Autodesk Fusion 360 part; units mm, degrees
(part 4 of 5)
  spline S564 degree 3 poles (63.6009, -62.117) (63.5452, -62.1873) (63.4918, -62.2601) (63.4399, -62.3343) (63.4147, -62.3703) (63.3907, -62.4074) (63.3664, -62.4443) (63.3253, -62.5068) (63.2844, -62.5696) (63.2459, -62.6346) (63.2219, -62.6752) (63.1997, -62.7175) (63.1767, -62.7591) (63.1472, -62.8123) (63.1177, -62.8655) (63.0898, -62.9203) (63.0665, -62.9662) (63.0447, -63.0135) (63.0226, -63.0606) (62.9975, -63.1139) (62.9727, -63.1675) (62.9491, -63.2223) (62.928, -63.2715) (62.9077, -63.3215) (62.8877, -63.3719) (62.8656, -63.4276) (62.8443, -63.4839) (62.8237, -63.541) (62.8052, -63.5925) (62.787, -63.6442) (62.7696, -63.6968) (62.75, -63.7563) (62.7315, -63.8169) (62.7134, -63.8779) (62.6978, -63.9304) (62.6821, -63.9828) (62.6676, -64.0364) (62.6498, -64.1023) (62.6337, -64.1699) (62.6177, -64.2374) (62.6055, -64.2884) (62.5926, -64.3387) (62.5815, -64.3906) (62.5635, -64.4745) (62.5478, -64.5606) (62.5323, -64.6468) knots 516 516 516 516 517 517 517 518 518 518 519 519 519 520 520 520 521 521 521 522 522 522 523 523 523 524 524 524 525 525 525 526 526 526 527 527 527 528 528 528 529 529 529 530 530 530 531 531 531 531
  spline S565 degree 3 poles (62.5323, -64.6468) (62.5253, -64.6848) (62.5171, -64.7216) (62.5105, -64.76) (62.4896, -64.8838) (62.4713, -65.0101) (62.4555, -65.1388) knots 531 531 531 531 532 532 532 533 533 533 533
  spline S566 degree 3 poles (62.4555, -65.1388) (62.4498, -65.1844) (62.4459, -65.2317) (62.4409, -65.2779) (62.4315, -65.3648) (62.4223, -65.4519) (62.4152, -65.541) (62.4107, -65.5971) (62.4076, -65.6547) (62.404, -65.7118) (62.4004, -65.769) (62.3956, -65.8251) (62.3929, -65.8832) knots 533 533 533 533 534 534 534 535 535 535 536 536 536 537 537 537 537
  spline S567 degree 3 poles (62.3929, -65.8832) (60.929, -65.0924) (59.2396, -64.7303) (57.6027, -64.3796) (57.0063, -64.2518) (56.4429, -64.1311) (55.8865, -63.9902) (53.8629, -63.4779) (52.3936, -62.8929) (51.1226, -62.0932) (50.698, -61.826) (50.2974, -61.5052) (49.8733, -61.1654) (49.4956, -60.8629) (49.1052, -60.5501) (48.6984, -60.2812) knots 537 537 537 537 538 538 538 539 539 539 540 540 540 541 541 541 542 542 542 542
  spline S568 degree 3 poles (48.6984, -60.2812) (48.112, -59.6879) (47.5333, -59.0646) (46.9735, -58.4616) (46.4472, -57.8948) (45.9032, -57.3085) (45.3521, -56.7472) (45.2642, -56.6576) (45.1756, -56.5693) (45.0868, -56.4809) knots 542 542 542 542 543 543 543 544 544 544 545 545 545 545
  line L80 (45.0868, -56.4809) -> (45.0182, -56.4139)
  spline S569 degree 3 poles (45.0182, -56.4139) (44.6949, -56.0962) (44.3697, -55.7813) (44.0447, -55.4664) (43.215, -54.6625) (42.357, -53.8314) (41.5512, -52.9714) knots 546 546 546 546 547 547 547 548 548 548 548
  line L81 (41.5512, -52.9714) -> (41.5003, -52.9185)
  spline S570 degree 3 poles (41.5003, -52.9185) (41.4832, -52.9013) (41.4663, -52.884) (41.4498, -52.8662) knots 549 549 549 549 550 550 550 550
  spline S571 degree 3 poles (41.4498, -52.8662) (40.8528, -52.2243) (40.2539, -51.5635) (39.6747, -50.9244) knots 550 550 550 550 551 551 551 551
  line L82 (39.6747, -50.9244) -> (39.2528, -50.4591)
  spline S572 degree 3 poles (39.2528, -50.4591) (39.2451, -50.451) (38.4952, -49.6609) (37.6236, -48.7686) knots 552 552 552 552 553 553 553 553
  line L83 (37.6236, -48.7686) -> (37.6335, -48.7479)
  spline S573 degree 3 poles (37.6335, -48.7479) (37.6362, -48.7422) (37.6387, -48.7366) (37.6415, -48.7309) knots 554 554 554 554 555 555 555 555
  line L84 (37.6415, -48.7309) -> (37.6464, -48.7205)
  spline S574 degree 3 poles (37.6464, -48.7205) (37.7592, -48.4837) (37.8712, -48.2488) (37.9778, -48.0153) knots 556 556 556 556 557 557 557 557
  spline S575 degree 3 poles (37.9778, -48.0153) (38.4446, -46.9908) (38.9842, -45.9631) (39.6279, -44.8736) (39.7256, -44.7081) (39.8268, -44.5413) (39.9304, -44.3732) (39.9626, -44.3209) (39.9966, -44.2678) (40.0294, -44.2152) (40.1022, -44.0987) (40.1756, -43.9818) (40.2514, -43.8637) (40.2926, -43.7995) (40.3355, -43.7343) (40.3776, -43.6696) (40.4483, -43.5611) (40.5196, -43.4521) (40.593, -43.342) (40.6394, -43.2723) (40.687, -43.2017) (40.7346, -43.1313) (40.8076, -43.0232) (40.8818, -42.9144) (40.9576, -42.8046) (41.0074, -42.7324) (41.0578, -42.6597) (41.1088, -42.5866) (41.1873, -42.4743) (41.2677, -42.3606) (41.3491, -42.2463) (41.4006, -42.1739) (41.452, -42.1016) (41.5048, -42.0282) (41.5924, -41.9065) (41.6829, -41.7827) (41.7741, -41.6583) (41.824, -41.5902) (41.8729, -41.5229) (41.9239, -41.4539) (42.0361, -41.3024) (42.152, -41.1479) (42.2696, -40.992) (42.3028, -40.9481) (42.3343, -40.9055) (42.3678, -40.8612) (42.3733, -40.854) (42.3793, -40.8464) (42.3847, -40.8392) knots 557 557 557 557 558 558 558 559 559 559 560 560 560 561 561 561 562 562 562 563 563 563 564 564 564 565 565 565 566 566 566 567 567 567 568 568 568 569 569 569 570 570 570 571 571 571 572 572 572 573 573 573 573
  spline S576 degree 3 poles (42.3847, -40.8392) (42.3816, -40.8575) (42.3797, -40.876) (42.3766, -40.8943) (42.3477, -41.0657) (42.3222, -41.2377) (42.301, -41.4103) knots 573 573 573 573 574 574 574 575 575 575 575
  spline S577 degree 3 poles (42.301, -41.4103) (42.2993, -41.4247) (42.297, -41.439) (42.2953, -41.4534) knots 575 575 575 575 576 576 576 576
  spline S578 degree 3 poles (42.2953, -41.4534) (42.2741, -41.632) (42.2583, -41.8113) (42.2454, -41.991) (42.243, -42.025) (42.2403, -42.059) (42.2381, -42.0931) (42.2272, -42.2674) (42.2204, -42.4419) (42.2172, -42.6167) (42.2166, -42.6524) (42.2164, -42.6881) (42.2161, -42.7238) knots 576 576 576 576 577 577 577 578 578 578 579 579 579 580 580 580 580
  spline S579 degree 3 poles (42.2161, -42.7238) (42.2146, -42.9023) (42.2161, -43.0809) (42.2227, -43.2596) (42.2235, -43.2795) (42.2249, -43.2994) (42.2257, -43.3194) knots 580 580 580 580 581 581 581 582 582 582 582
  spline S580 degree 3 poles (42.2257, -43.3194) (42.233, -43.491) (42.2442, -43.6625) (42.2589, -43.8339) (42.2612, -43.8603) (42.2629, -43.8868) (42.2654, -43.9132) (42.2817, -44.0896) (42.3029, -44.2657) (42.3272, -44.4415) (42.3323, -44.4781) (42.3374, -44.5148) (42.3428, -44.5514) (42.3687, -44.726) (42.3981, -44.9001) (42.4318, -45.0736) (42.4377, -45.1045) (42.4444, -45.1352) (42.4506, -45.166) knots 582 582 582 582 583 583 583 584 584 584 585 585 585 586 586 586 587 587 587 588 588 588 588
  spline S581 degree 3 poles (42.4506, -45.166) (42.4876, -45.3485) (42.5276, -45.5306) (42.5733, -45.7116) knots 588 588 588 588 589 589 589 589
  ellipse E72 centre (56.6932, -41.7046) end of major axis (43.7029, -48.5965) minor radius 14.1081 (42.5733, -45.7116) -> (43.5329, -48.2653) ccw
  line L85 (43.5329, -48.2653) -> (43.592, -48.3797)
  ellipse E73 centre (53.8644, -44.6888) end of major axis (43.8869, -37.796) minor radius 10.4203 (43.592, -48.3797) -> (45.426, -51.0359) ccw
  spline S582 degree 3 poles (45.426, -51.0359) (49.4743, -55.6013) (55.686, -55.4114) (59.19, -54.8409) knots 592 592 592 592 593 593 593 593
  ellipse E74 centre (57.3687, -53.9917) end of major axis (58.3854, -55.9418) minor radius 1.7755 (58.8424, -55.5685) -> (59.19, -54.8409) ccw
  spline S583 degree 3 poles (58.8424, -55.5685) (58.7415, -55.6913) (58.4247, -56.1135) (58.5847, -56.3946) knots 594 594 594 594 595 595 595 595
  spline S584 degree 3 poles (58.5847, -56.3946) (58.6701, -56.545) (58.8483, -56.6007) (59.1137, -56.5599) (59.6558, -56.4764) (60.4864, -55.9417) (60.6187, -55.8147) knots 595 595 595 595 596 596 596 597 597 597 597
  spline S585 degree 3 poles (60.6187, -55.8147) (60.6941, -55.7415) (60.7615, -55.6603) (60.8219, -55.569) knots 597 597 597 597 598 598 598 598
  spline S586 degree 3 poles (60.8219, -55.569) (61.9106, -56.1881) (63.4433, -56.428) (64.404, -55.5311) knots 598 598 598 598 599 599 599 599
  spline S587 degree 3 poles (64.404, -55.5311) (64.5308, -55.413) (64.5814, -55.2388) (64.5394, -55.065) (64.4963, -54.8868) (64.3637, -54.7461) (64.1931, -54.6977) knots 599 599 599 599 600 600 600 601 601 601 601
  line L86 (64.1931, -54.6977) -> (64.1043, -54.6725)
  spline S588 degree 3 poles (64.1043, -54.6725) (63.4425, -54.485) (62.8117, -54.3065) (62.2722, -53.9865) knots 602 602 602 602 603 603 603 603
  spline S589 degree 3 poles (62.2722, -53.9865) (65.482, -52.7483) (70.6811, -49.8991) (71.9549, -44.1657) knots 603 603 603 603 604 604 604 604
  ellipse E75 centre (60.8257, -42.7322) end of major axis (67.3496, -31.9795) minor radius 11.0029 (71.9549, -44.1657) -> (72.2688, -40.9515) ccw
  line L87 (72.2688, -40.9515) -> (72.2641, -40.8116)
  ellipse E76 centre (64.0549, -39.8245) end of major axis (61.025, -29.7414) minor radius 7.9821 (72.2641, -40.8116) -> (71.864, -38.1233) ccw
  spline S590 degree 3 poles (71.864, -38.1233) (71.3093, -36.0365) (70.2055, -34.159) (68.6718, -32.6934) (66.8596, -30.9618) (64.5325, -29.8716) (61.9419, -29.5414) (61.4484, -29.4785) (60.9282, -29.4355) (60.3894, -29.4131) knots 607 607 607 607 608 608 608 609 609 609 610 610 610 610
  spline S591 degree 3 poles (60.3894, -29.4131) (62.1442, -28.8512) (63.6979, -28.4325) (65.1254, -28.1369) (66.5537, -27.841) (67.8818, -27.634) (69.1854, -27.505) (69.4822, -27.4757) (69.783, -27.4409) (70.086, -27.4058) (70.2077, -27.3917) (70.33, -27.3777) (70.4526, -27.3638) (70.5356, -27.3544) (70.6189, -27.3455) (70.7022, -27.3365) (70.7407, -27.3324) (70.779, -27.328) (70.8175, -27.3239) (71.0588, -27.2986) (71.3009, -27.2759) (71.5425, -27.2581) knots 610 610 610 610 611 611 611 612 612 612 613 613 613 614 614 614 615 615 615 616 616 616 617 617 617 617
  spline S592 degree 3 poles (71.5425, -27.2581) (71.546, -27.2578) (71.5495, -27.2575) (71.5529, -27.2572) knots 617 617 617 617 618 618 618 618
  spline S593 degree 3 poles (71.5529, -27.2572) (71.6573, -27.2496) (71.7614, -27.2435) (71.8655, -27.238) (71.8846, -27.237) (71.9037, -27.2355) (71.9227, -27.2346) (72.011, -27.2303) (72.0988, -27.2279) (72.1867, -27.2255) (72.222, -27.2245) (72.2575, -27.2227) (72.2928, -27.2221) (72.3654, -27.2208) (72.4375, -27.2216) (72.5098, -27.2218) (72.5604, -27.2219) (72.6112, -27.2211) (72.6617, -27.222) (72.7198, -27.2231) (72.7774, -27.2263) (72.8352, -27.2286) (72.8911, -27.2307) (72.9472, -27.2324) (73.0028, -27.2357) knots 618 618 618 618 619 619 619 620 620 620 621 621 621 622 622 622 623 623 623 624 624 624 625 625 625 626 626 626 626
  spline S594 degree 3 poles (73.0028, -27.2357) (73.1238, -27.2975) (73.2558, -27.3369) (73.3903, -27.3647) knots 626 626 626 626 627 627 627 627
  spline S595 degree 3 poles (73.3903, -27.3647) (73.3976, -27.3661) (73.4048, -27.3679) (73.412, -27.3693) knots 627 627 627 627 628 628 628 628
  spline S596 degree 3 poles (73.412, -27.3693) (73.4649, -27.3796) (73.5178, -27.3883) (73.5709, -27.3953) (73.5825, -27.3968) (73.594, -27.3989) (73.6056, -27.4003) (73.6624, -27.4071) (73.719, -27.4127) (73.7748, -27.417) (74.7297, -27.4916) (75.7369, -27.313) (76.5412, -26.9278) (77.045, -26.6866) (77.529, -26.3489) (77.9038, -25.9766) (78.1899, -25.6923) (78.1926, -25.1937) (77.9094, -24.8875) knots 628 628 628 628 629 629 629 630 630 630 631 631 631 632 632 632 633 633 633 634 634 634 634
  spline S597 degree 3 poles (77.9094, -24.8875) (77.5689, -24.5207) (77.0072, -24.5165) (76.597, -24.5137) (76.5457, -24.5133) (76.4961, -24.513) (76.4487, -24.5119) knots 634 634 634 634 635 635 635 636 636 636 636
  spline S598 degree 3 poles (76.4487, -24.5119) (76.366, -24.5102) (76.283, -24.5097) (76.1996, -24.509) knots 636 636 636 636 637 637 637 637
  spline S599 degree 3 poles (76.1996, -24.509) (75.7309, -24.5056) (75.2883, -24.5023) (74.8824, -24.3113) (74.8326, -24.2878) (74.8004, -24.2682) (74.7801, -24.2534) knots 637 637 637 637 638 638 638 639 639 639 639
  spline S600 degree 3 poles (74.7801, -24.2534) (74.8118, -24.232) (74.8678, -24.2024) (74.9585, -24.171) (75.4633, -23.9965) (75.9971, -24.0882) (76.4053, -24.1876) (76.515, -24.2143) (76.6253, -24.2575) (76.7421, -24.3032) (76.9584, -24.3877) (77.1762, -24.4768) (77.4332, -24.4704) knots 639 639 639 639 640 640 640 641 641 641 642 642 642 643 643 643 643
  spline S601 degree 3 poles (77.4332, -24.4704) (77.6931, -24.4651) (77.9655, -24.3065) (78.0953, -24.0844) (78.2126, -23.8837) (78.2118, -23.6512) (78.0931, -23.4295) (77.584, -22.4789) (76.7066, -22.0668) (75.9993, -21.8141) (75.9082, -21.7815) (75.8143, -21.7464) (75.718, -21.7106) (75.6611, -21.6894) (75.6027, -21.6677) (75.5439, -21.646) knots 643 643 643 643 644 644 644 645 645 645 646 646 646 647 647 647 648 648 648 648
  spline S602 degree 3 poles (75.5439, -21.646) (75.5305, -21.6411) (75.5172, -21.6363) (75.5037, -21.6314) (75.4494, -21.6115) (75.3942, -21.5917) (75.3384, -21.5721) (75.3288, -21.5687) (75.3194, -21.5654) (75.3098, -21.562) knots 648 648 648 648 649 649 649 650 650 650 651 651 651 651
  spline S603 degree 3 poles (75.3098, -21.562) (75.2458, -21.5398) (75.181, -21.5181) (75.1155, -21.4971) (75.1056, -21.4939) (75.0956, -21.491) (75.0856, -21.4878) (75.0302, -21.4704) (74.9744, -21.4537) (74.9181, -21.4377) (74.9031, -21.4335) (74.8881, -21.4292) (74.873, -21.4251) (74.7411, -21.3889) (74.6074, -21.3581) (74.473, -21.3352) (74.4574, -21.3326) (74.4419, -21.3303) (74.4264, -21.3279) (74.3698, -21.3191) (74.3132, -21.3119) (74.2567, -21.3064) (74.2447, -21.3052) (74.2327, -21.3036) (74.2207, -21.3026) (74.1534, -21.2969) (74.0861, -21.2937) (74.019, -21.2935) (74.0157, -21.2935) (74.0124, -21.293) (74.0091, -21.293) (73.9985, -21.293) (73.9881, -21.2942) (73.9775, -21.2944) (73.9331, -21.295) (73.8887, -21.2967) (73.8445, -21.3001) (73.8254, -21.3015) (73.8063, -21.3036) (73.7872, -21.3056) (73.7475, -21.3098) (73.708, -21.3152) (73.6687, -21.3218) (73.6485, -21.3252) (73.6284, -21.3286) (73.6083, -21.3327) (73.5685, -21.3408) (73.5288, -21.3508) (73.4893, -21.3617) (73.4713, -21.3667) (73.4531, -21.3709) (73.4351, -21.3765) (73.3817, -21.3932) (73.3287, -21.4123) (73.2763, -21.4347) (73.2732, -21.436) (73.2701, -21.4367) (73.267, -21.4381) knots 651 651 651 651 652 652 652 653 653 653 654 654 654 655 655 655 656 656 656 657 657 657 658 658 658 659 659 659 660 660 660 661 661 661 662 662 662 663 663 663 664 664 664 665 665 665 666 666 666 667 667 667 668 668 668 669 669 669 670 670 670 670
  spline S604 degree 3 poles (73.267, -21.4381) (73.2211, -21.4583) (73.1773, -21.4804) (73.1351, -21.5046) knots 670 670 670 670 671 671 671 671
  spline S605 degree 3 poles (73.1351, -21.5046) (73.0842, -21.4915) (73.0305, -21.4797) (72.9785, -21.4671) (72.9191, -21.4527) (72.8604, -21.438) (72.7996, -21.4243) (72.734, -21.4096) (72.6664, -21.396) (72.5992, -21.3821) (72.5352, -21.3688) (72.4719, -21.3552) (72.4066, -21.3428) (72.3399, -21.33) (72.2713, -21.3184) (72.2032, -21.3064) (72.1348, -21.2944) (72.0669, -21.282) (71.9971, -21.2708) (71.9297, -21.2599) (71.8604, -21.2501) (71.7917, -21.2399) (71.7184, -21.2291) (71.6457, -21.2179) (71.571, -21.2079) (71.5034, -21.1988) (71.4341, -21.1908) (71.3654, -21.1823) (71.2874, -21.1727) (71.2098, -21.1629) (71.1304, -21.1541) (71.0627, -21.1466) (70.9934, -21.1401) (70.9247, -21.1333) (70.8419, -21.125) (70.7595, -21.1164) (70.6753, -21.109) (70.6076, -21.103) (70.5382, -21.0979) (70.4696, -21.0925) (70.3826, -21.0855) (70.296, -21.0784) (70.2078, -21.0723) (70.1399, -21.0677) (70.0707, -21.0639) (70.0021, -21.0598) (69.9107, -21.0543) (69.8196, -21.0485) (69.7269, -21.0438) (69.6603, -21.0405) (69.5923, -21.038) (69.525, -21.0351) (69.4287, -21.0309) (69.3327, -21.0265) (69.2351, -21.0233) (69.1686, -21.021) (69.101, -21.0196) (69.0339, -21.0178) (68.934, -21.0151) (68.8344, -21.0122) (68.7333, -21.0104) (68.6667, -21.0092) (68.5991, -21.0088) (68.532, -21.008) (68.4289, -21.0067) (68.326, -21.0053) (68.2218, -21.0049) (68.1555, -21.0046) (68.0882, -21.0052) (68.0215, -21.0053) (67.915, -21.0055) (67.8086, -21.0055) (67.7011, -21.0066) (67.6353, -21.0072) (67.5687, -21.0086) (67.5026, -21.0096) (67.3931, -21.0112) (67.2838, -21.0126) (67.1733, -21.0151) (67.1074, -21.0166) (67.0408, -21.0188) (66.9746, -21.0206) (66.8626, -21.0236) (66.7507, -21.0264) (66.6379, -21.0303) (66.5728, -21.0325) (66.5071, -21.0354) (66.4418, -21.0379) (66.3271, -21.0423) (66.2126, -21.0466) (66.0972, -21.0518) (66.0317, -21.0548) (65.9656, -21.0584) (65.8998, -21.0616) (65.7836, -21.0673) (65.6675, -21.0729) (65.5507, -21.0794) (65.4858, -21.0831) (65.4205, -21.0873) (65.3554, -21.0912) (65.2373, -21.0982) (65.1192, -21.1051) (65.0005, -21.1129) (64.9342, -21.1173) (64.8675, -21.1223) (64.801, -21.1269) (64.6832, -21.1351) (64.5654, -21.1431) (64.4472, -21.152) (64.3812, -21.1569) (64.315, -21.1625) (64.2489, -21.1677) (64.1292, -21.1771) (64.0096, -21.1864) (63.8897, -21.1965) (63.8234, -21.2021) (63.7569, -21.2083) (63.6905, -21.2141) (63.5718, -21.2245) (63.4531, -21.2347) (63.3343, -21.2458) (63.2606, -21.2527) (63.1868, -21.2601) (63.1131, -21.2673) (63.0004, -21.2781) (62.8878, -21.2888) (62.7751, -21.3002) (62.7033, -21.3075) (62.6315, -21.3154) (62.5597, -21.3229) (62.4451, -21.3349) (62.3305, -21.3467) (62.216, -21.3592) (62.1434, -21.3672) (62.071, -21.3757) (61.9984, -21.3838) (61.8854, -21.3966) (61.7724, -21.4091) (61.6596, -21.4224) (61.5783, -21.4319) (61.4974, -21.442) (61.4162, -21.4518) (61.3125, -21.4643) (61.2087, -21.4766) (61.1052, -21.4895) (61.0166, -21.5006) (60.9284, -21.5123) (60.8401, -21.5236) (60.7441, -21.536) (60.648, -21.548) (60.5523, -21.5607) (60.4622, -21.5727) (60.3727, -21.5851) (60.2829, -21.5973) (60.1895, -21.61) (60.0958, -21.6225) (60.0028, -21.6355) (59.9108, -21.6484) (59.8195, -21.6617) (59.7279, -21.6749) (59.6379, -21.6878) (59.5475, -21.7004) (59.4579, -21.7136) (59.3548, -21.7288) (59.2526, -21.7444) (59.1501, -21.7599) (59.0734, -21.7715) (58.9962, -21.7828) (58.9199, -21.7945) (58.8058, -21.8121) (58.6929, -21.8302) (58.5798, -21.8481) (58.5154, -21.8583) (58.4503, -21.8683) (58.3862, -21.8786) (58.2765, -21.8963) (58.1682, -21.9144) (58.0595, -21.9324) (57.9929, -21.9434) (57.9256, -21.9542) (57.8593, -21.9653) (57.7345, -21.9863) (57.6112, -22.0077) (57.4879, -22.0291) (57.4394, -22.0375) (57.3901, -22.0457) (57.3419, -22.0541) (57.1705, -22.0842) (57.0007, -22.1145) (56.8325, -22.1452) knots 671 671 671 671 672 672 672 673 673 673 674 674 674 675 675 675 676 676 676 677 677 677 678 678 678 679 679 679 680 680 680 681 681 681 682 682 682 683 683 683 684 684 684 685 685 685 686 686 686 687 687 687 688 688 688 689 689 689 690 690 690 691 691 691 692 692 692 693 693 693 694 694 694 695 695 695 696 696 696 697 697 697 698 698 698 699 699 699 700 700 700 701 701 701 702 702 702 703 703 703 704 704 704 705 705 705 706 706 706 707 707 707 708 708 708 709 709 709 710 710 710 711 711 711 712 712 712 713 713 713 714 714 714 715 715 715 716 716 716 717 717 717 718 718 718 719 719 719 720 720 720 721 721 721 722 722 722 723 723 723 724 724 724 725 725 725 726 726 726 727 727 727 728 728 728 729 729 729 730 730 730 731 731 731 732 732 732 733 733 733 734 734 734 734
  spline S606 degree 3 poles (56.8325, -22.1452) (56.7516, -22.0203) (56.6697, -21.8961) (56.5871, -21.7727) (54.8757, -19.2194) (52.3141, -16.9233) (48.9732, -14.9485) knots 734 734 734 734 735 735 735 736 736 736 736
  spline S607 degree 3 poles (48.9732, -14.9485) (48.5872, -14.7198) (48.1976, -14.5051) (47.805, -14.3045) (47.6332, -14.2167) (47.4608, -14.1317) (47.2879, -14.0494) (44.6941, -12.8144) (41.9778, -12.1891) (39.2765, -12.1892) (37.318, -12.1892) (35.3671, -12.5176) (33.4774, -13.1814) (30.9108, -14.0828) (28.7605, -15.695) (27.423, -17.7205) (27.3252, -17.8685) (27.2307, -18.0215) (27.1393, -18.1789) (27.0921, -18.2604) (27.0482, -18.3463) (27.0027, -18.4301) (26.9604, -18.5081) (26.9164, -18.584) (26.8757, -18.664) (26.8225, -18.7685) (26.773, -18.8774) (26.7226, -18.9851) (26.6927, -19.0488) (26.661, -19.1104) (26.6322, -19.1752) (26.5916, -19.2663) (26.5547, -19.3609) (26.5162, -19.454) (26.4815, -19.538) (26.4448, -19.6199) (26.4116, -19.7055) knots 736 736 736 736 737 737 737 738 738 738 739 739 739 740 740 740 741 741 741 742 742 742 743 743 743 744 744 744 745 745 745 746 746 746 747 747 747 748 748 748 748
  spline S608 degree 3 poles (26.4116, -19.7055) (26.2671, -19.9176) (26.124, -20.1312) (25.9808, -20.3449) (25.4407, -21.1516) (24.882, -21.9858) (24.2507, -22.7084) knots 748 748 748 748 749 749 749 750 750 750 750
  spline S609 degree 3 poles (24.2507, -22.7084) (23.9887, -23.009) (23.7265, -23.3073) (23.4649, -23.6048) (22.1621, -25.0863) (20.8153, -26.6186) (19.6453, -28.2909) knots 750 750 750 750 751 751 751 752 752 752 752
  spline S610 degree 3 poles (19.6453, -28.2909) (19.5404, -28.441) (19.4379, -28.5893) (19.3374, -28.7361) (19.3091, -28.7774) (19.2822, -28.8176) (19.2543, -28.8587) (19.1834, -28.9629) (19.1126, -29.067) (19.0439, -29.1697) (19.0087, -29.2222) (18.9749, -29.2739) (18.9402, -29.326) (18.8806, -29.4159) (18.8208, -29.5058) (18.7629, -29.5944) (18.7254, -29.6518) (18.6891, -29.7084) (18.6522, -29.7653) (18.5995, -29.8469) (18.5467, -29.9284) (18.4952, -30.009) knots 752 752 752 752 753 753 753 754 754 754 755 755 755 756 756 756 757 757 757 758 758 758 759 759 759 759
  spline S611 degree 3 poles (18.4952, -30.009) (18.4562, -30.0703) (18.4183, -30.1308) (18.38, -30.1916) (18.3328, -30.2665) (18.2856, -30.3414) (18.2396, -30.4156) (18.2003, -30.479) (18.1618, -30.5418) (18.1233, -30.6046) (18.0801, -30.6752) (18.037, -30.7458) (17.9948, -30.8158) (17.956, -30.8801) (17.918, -30.944) (17.88, -31.0079) (17.8401, -31.0751) (17.8002, -31.1424) (17.7612, -31.2091) (17.7233, -31.2739) (17.686, -31.3384) (17.649, -31.4027) (17.6281, -31.439) (17.6063, -31.4758) (17.5857, -31.5119) knots 759 759 759 759 760 760 760 761 761 761 762 762 762 763 763 763 764 764 764 765 765 765 766 766 766 767 767 767 767
  spline S612 degree 3 poles (17.5857, -31.5119) (17.5359, -31.4729) (17.4863, -31.4335) (17.4365, -31.3935) knots 767 767 767 767 768 768 768 768
  line L88 (17.4365, -31.3935) -> (17.39, -31.3561)
  spline S613 degree 3 poles (17.39, -31.3561) (17.3009, -31.2841) (17.2122, -31.2118) (17.124, -31.1375) knots 769 769 769 769 770 770 770 770
  spline S614 degree 3 poles (17.124, -31.1375) (17.084, -31.1043) (17.0441, -31.0695) (17.0036, -31.0342) knots 770 770 770 770 771 771 771 771
  line L89 (17.0036, -31.0342) -> (16.95, -30.9885)
  spline S615 degree 3 poles (16.95, -30.9885) (16.9018, -30.9476) (16.8536, -30.9064) (16.8057, -30.864) knots 772 772 772 772 773 773 773 773
  spline S616 degree 3 poles (16.8057, -30.864) (16.697, -30.7682) (16.5886, -30.67) (16.4808, -30.5693) knots 773 773 773 773 774 774 774 774
  spline S617 degree 3 poles (16.4808, -30.5693) (16.3988, -30.4925) (16.3129, -30.4111) (16.2238, -30.3266) (15.2069, -29.3613) (13.8119, -28.0392) (12.3706, -28.2063) knots 774 774 774 774 775 775 775 776 776 776 776
  spline S618 degree 3 poles (12.3706, -28.2063) (11.3121, -28.3276) (10.6648, -29.6666) (10.192, -30.644) (10.1146, -30.8039) (10.0435, -30.9512) (9.9773, -31.0774) knots 776 776 776 776 777 777 777 778 778 778 778
  ellipse E77 centre (11.8632, -31.7575) end of major axis (13.4861, -29.4742) minor radius 1.9679 (9.9773, -31.0774) -> (9.7069, -31.7449) ccw
  spline S619 degree 3 poles (9.7069, -31.7449) (9.033, -33.0747) (8.8594, -34.1568) (9.1607, -35.1495) knots 779 779 779 779 780 780 780 780
  spline S620 degree 3 poles (48.123, -20.7251) (48.3208, -20.8706) (48.5228, -21.0158) (48.6823, -21.1437) knots 0 0 0 0 1 1 1 1
  spline S621 degree 3 poles (48.6823, -21.1437) (48.8433, -21.2712) (48.961, -21.3799) (49.0283, -21.4385) knots 1 1 1 1 2 2 2 2
  spline S622 degree 3 poles (49.0283, -21.4385) (49.1643, -21.5553) (49.2965, -21.626) (49.4332, -21.6748) knots 2 2 2 2 3 3 3 3
  spline S623 degree 3 poles (49.4332, -21.6748) (49.5699, -21.7203) (49.716, -21.7493) (49.8473, -21.6975) knots 3 3 3 3 4 4 4 4
  spline S624 degree 3 poles (49.8473, -21.6975) (49.9756, -21.6472) (50.0605, -21.5026) (50.0417, -21.2966) knots 4 4 4 4 5 5 5 5
  spline S625 degree 3 poles (50.0417, -21.2966) (50.0259, -21.0922) (49.8947, -20.8452) (49.6877, -20.6694) knots 5 5 5 5 6 6 6 6
  spline S626 degree 3 poles (49.6877, -20.6694) (49.5849, -20.5802) (49.3943, -20.4536) (49.1673, -20.3464) knots 6 6 6 6 7 7 7 7
  spline S627 degree 3 poles (49.1673, -20.3464) (48.9403, -20.2377) (48.679, -20.1467) (48.4336, -20.0797) knots 7 7 7 7 8 8 8 8
  spline S628 degree 3 poles (48.4336, -20.0797) (47.9407, -19.9524) (47.5203, -19.8779) (47.4482, -19.9917) knots 8 8 8 8 9 9 9 9
  spline S629 degree 3 poles (47.4482, -19.9917) (47.3708, -20.1159) (47.724, -20.4398) (48.123, -20.7251) knots 9 9 9 9 10 10 10 10
  spline S630 degree 3 poles (54.519, -26.2828) (54.6474, -26.552) (54.7243, -26.7777) (54.7654, -26.9025) knots 0 0 0 0 1 1 1 1
  spline S631 degree 3 poles (54.7654, -26.9025) (54.8508, -27.1552) (54.9222, -27.3429) (54.9884, -27.4995) knots 1 1 1 1 2 2 2 2
  spline S632 degree 3 poles (54.9884, -27.4995) (55.0576, -27.6528) (55.1102, -27.8097) (55.2317, -27.8818) knots 2 2 2 2 3 3 3 3
  spline S633 degree 3 poles (55.2317, -27.8818) (55.3466, -27.9525) (55.5538, -27.8842) (55.6953, -27.6157) knots 3 3 3 3 4 4 4 4
  spline S634 degree 3 poles (55.6953, -27.6157) (55.8378, -27.3525) (55.8521, -26.94) (55.7257, -26.5798) knots 4 4 4 4 5 5 5 5
  spline S635 degree 3 poles (55.7257, -26.5798) (55.6656, -26.3966) (55.528, -26.1062) (55.3254, -25.8125) knots 5 5 5 5 6 6 6 6
  ellipse E78 centre (54.5419, -25.579) end of major axis (53.4603, -24.3926) minor radius 0.4686 (55.3254, -25.8125) -> (54.5895, -24.9605) ccw
  spline S636 degree 3 poles (54.5895, -24.9605) (54.0491, -24.4428) (53.4487, -24.1366) (53.3658, -24.2566) knots 7 7 7 7 8 8 8 8
  spline S637 degree 3 poles (53.3658, -24.2566) (53.2884, -24.3662) (53.6834, -24.8362) (54.0388, -25.4185) knots 8 8 8 8 9 9 9 9
  ellipse E79 centre (53.8321, -25.5333) end of major axis (54.6696, -26.8641) minor radius 0.236 (54.519, -26.2828) -> (54.0388, -25.4185) ccw
  spline S638 degree 3 poles (50.8598, -27.2408) (50.9671, -27.4549) (51.0414, -27.6309) (51.0863, -27.7297) knots 0 0 0 0 1 1 1 1
  spline S639 degree 3 poles (51.0863, -27.7297) (51.1758, -27.9267) (51.2795, -28.0797) (51.3901, -28.2001) knots 1 1 1 1 2 2 2 2
  spline S640 degree 3 poles (51.3901, -28.2001) (51.5018, -28.3177) (51.6253, -28.4126) (51.7665, -28.4147) knots 2 2 2 2 3 3 3 3
  spline S641 degree 3 poles (51.7665, -28.4147) (51.9044, -28.4174) (52.0376, -28.3024) (52.0976, -28.0875) knots 3 3 3 3 4 4 4 4
  spline S642 degree 3 poles (52.0976, -28.0875) (52.1593, -27.8749) (52.1313, -27.5776) (52.0072, -27.3082) knots 4 4 4 4 5 5 5 5
  spline S643 degree 3 poles (52.0072, -27.3082) (51.946, -27.1729) (51.8181, -26.9567) (51.6452, -26.7373) knots 5 5 5 5 6 6 6 6
  spline S644 degree 3 poles (51.6452, -26.7373) (51.4732, -26.5157) (51.2593, -26.2885) (51.0473, -26.0924) knots 6 6 6 6 7 7 7 7
  spline S645 degree 3 poles (51.0473, -26.0924) (50.6199, -25.7035) (50.2253, -25.4062) (50.1137, -25.4826) knots 7 7 7 7 8 8 8 8
  spline S646 degree 3 poles (50.1137, -25.4826) (49.9947, -25.5652) (50.2121, -26.0472) (50.4829, -26.5331) knots 8 8 8 8 9 9 9 9
  spline S647 degree 3 poles (50.4829, -26.5331) (50.6161, -26.7777) (50.7535, -27.0271) (50.8598, -27.2408) knots 9 9 9 9 10 10 10 10
  spline S648 degree 3 poles (35.606, -26.5164) (36.0331, -26.734) (36.4758, -26.945) (36.6494, -27.025) knots 0 0 0 0 1 1 1 1
  ellipse E80 centre (36.7803, -25.9398) end of major axis (36.0164, -24.9115) minor radius 0.9578 (36.6494, -27.025) -> (37.1596, -27.1121) ccw
  spline S649 degree 3 poles (37.1596, -27.1121) (37.3149, -27.0962) (37.4538, -27.0385) (37.5324, -26.922) knots 2 2 2 2 3 3 3 3
  ellipse E81 centre (36.9506, -26.5698) end of major axis (36.3535, -26.2427) minor radius 0.4632 (37.5324, -26.922) -> (37.5186, -26.4924) ccw
  spline S650 degree 3 poles (37.5186, -26.4924) (37.4321, -26.3358) (37.2616, -26.1831) (37.045, -26.0924) knots 4 4 4 4 5 5 5 5
  spline S651 degree 3 poles (37.045, -26.0924) (36.8278, -25.9933) (36.2822, -25.8688) (35.8095, -25.8296) knots 5 5 5 5 6 6 6 6
  spline S652 degree 3 poles (35.8095, -25.8296) (35.3354, -25.7889) (34.916, -25.7802) (34.8667, -25.9092) knots 6 6 6 6 7 7 7 7
  spline S653 degree 3 poles (34.8667, -25.9092) (34.8165, -26.0415) (35.1812, -26.2996) (35.606, -26.5164) knots 7 7 7 7 8 8 8 8
  ellipse E82 centre (39.9104, -20.7707) end of major axis (38.979, -20.3868) minor radius 0.2405 (40.5083, -20.8018) -> (39.8918, -20.5048) ccw
  spline S654 degree 3 poles (40.5083, -20.8018) (40.682, -20.9071) (40.8127, -21.0104) (40.891, -21.0676) knots 1 1 1 1 2 2 2 2
  ellipse E83 centre (41.162, -19.6978) end of major axis (40.3198, -18.1381) minor radius 1.1194 (40.891, -21.0676) -> (41.3687, -21.3065) ccw
  ellipse E84 centre (38.7915, -17.0558) end of major axis (35.7858, -12.8403) minor radius 1.2802 (41.3687, -21.3065) -> (41.7973, -21.2712) ccw
  spline S655 degree 3 poles (41.7973, -21.2712) (41.9101, -21.1907) (41.9565, -21.0326) (41.9097, -20.8377) knots 4 4 4 4 5 5 5 5
  spline S656 degree 3 poles (41.9097, -20.8377) (41.8644, -20.644) (41.7185, -20.4156) (41.4854, -20.2473) knots 5 5 5 5 6 6 6 6
  spline S657 degree 3 poles (41.4854, -20.2473) (41.3705, -20.1632) (41.1551, -20.0395) (40.8876, -19.9491) knots 6 6 6 6 7 7 7 7
  ellipse E85 centre (40.3401, -20.2534) end of major axis (39.2284, -20.0854) minor radius 0.4264 (40.8876, -19.9491) -> (40.0159, -19.7997) ccw
  spline S658 degree 3 poles (40.0159, -19.7997) (39.4304, -19.7905) (38.9618, -19.9626) (38.9719, -20.0982) knots 8 8 8 8 9 9 9 9
  spline S659 degree 3 poles (38.9719, -20.0982) (38.9795, -20.2395) (39.4438, -20.3308) (39.8918, -20.5048) knots 9 9 9 9 10 10 10 10
  spline S660 degree 3 poles (32.9683, -21.2796) (32.7639, -21.3481) (32.2874, -21.5778) (31.893, -21.8601) knots 0 0 0 0 1 1 1 1
  spline S661 degree 3 poles (31.893, -21.8601) (31.4932, -22.134) (31.2013, -22.4915) (31.295, -22.604) knots 1 1 1 1 2 2 2 2
  spline S662 degree 3 poles (31.295, -22.604) (31.3812, -22.7076) (31.7548, -22.6019) (32.1909, -22.5109) knots 2 2 2 2 3 3 3 3
  spline S663 degree 3 poles (32.1909, -22.5109) (32.6236, -22.4127) (33.1043, -22.3023) (33.295, -22.2382) knots 3 3 3 3 4 4 4 4
  spline S664 degree 3 poles (33.295, -22.2382) (33.6761, -22.1071) (33.918, -21.8083) (33.8539, -21.5376) knots 4 4 4 4 5 5 5 5
  spline S665 degree 3 poles (33.8539, -21.5376) (33.789, -21.2637) (33.3766, -21.1386) (32.9683, -21.2796) knots 5 5 5 5 6 6 6 6
  spline S666 degree 3 poles (32.1808, -17.5897) (32.404, -17.5415) (32.6302, -17.4957) (32.819, -17.4691) knots 0 0 0 0 1 1 1 1
  spline S667 degree 3 poles (32.819, -17.4691) (33.0085, -17.4406) (33.16, -17.431) (33.2462, -17.4212) knots 1 1 1 1 2 2 2 2
  spline S668 degree 3 poles (33.2462, -17.4212) (33.4182, -17.4002) (33.5665, -17.3487) (33.6948, -17.2712) knots 2 2 2 2 3 3 3 3
  ellipse E86 centre (26.4354, -15.3174) end of major axis (18.9091, -13.6868) minor radius 1.6767 (33.6948, -17.2712) -> (33.9605, -16.9529) ccw
  spline S669 degree 3 poles (33.9605, -16.9529) (33.9918, -16.8179) (33.9301, -16.6706) (33.7768, -16.5598) knots 4 4 4 4 5 5 5 5
  spline S670 degree 3 poles (33.7768, -16.5598) (33.6261, -16.4491) (33.3824, -16.3841) (33.1284, -16.4152) knots 5 5 5 5 6 6 6 6
  spline S671 degree 3 poles (33.1284, -16.4152) (33.0013, -16.4293) (32.7877, -16.4793) (32.562, -16.5715) knots 6 6 6 6 7 7 7 7
  ellipse E87 centre (32.2566, -17.0798) end of major axis (31.3112, -17.6424) minor radius 0.3189 (32.562, -16.5715) -> (31.8927, -16.9341) ccw
  spline S672 degree 3 poles (31.8927, -16.9341) (31.4828, -17.2179) (31.1821, -17.5223) (31.2417, -17.646) knots 8 8 8 8 9 9 9 9
  spline S673 degree 3 poles (31.2417, -17.646) (31.3032, -17.7741) (31.7352, -17.6885) (32.1808, -17.5897) knots 9 9 9 9 10 10 10 10
  spline S674 degree 3 poles (41.0641, -17.1583) (41.5838, -17.3508) (42.115, -17.5855) (42.3267, -17.6801) knots 0 0 0 0 1 1 1 1
  ellipse E88 centre (42.2817, -16.7801) end of major axis (41.1296, -15.9612) minor radius 0.7701 (42.3267, -17.6801) -> (42.9317, -17.8119) ccw
  spline S675 degree 3 poles (42.9317, -17.8119) (43.1112, -17.81) (43.2648, -17.7621) (43.3433, -17.646) knots 2 2 2 2 3 3 3 3
  ellipse E89 centre (42.6882, -17.2376) end of major axis (42.0249, -16.842) minor radius 0.4526 (43.3433, -17.646) -> (43.2908, -17.1921) ccw
  spline S676 degree 3 poles (43.2908, -17.1921) (43.1798, -17.0212) (42.9734, -16.8505) (42.7132, -16.744) knots 4 4 4 4 5 5 5 5
  spline S677 degree 3 poles (42.7132, -16.744) (42.4541, -16.6281) (41.791, -16.473) (41.2063, -16.4566) knots 5 5 5 5 6 6 6 6
  spline S678 degree 3 poles (41.2063, -16.4566) (40.6202, -16.4323) (40.1113, -16.4964) (40.0913, -16.6332) knots 6 6 6 6 7 7 7 7
  spline S679 degree 3 poles (40.0913, -16.6332) (40.0707, -16.773) (40.5487, -16.9613) (41.0641, -17.1583) knots 7 7 7 7 8 8 8 8
  ellipse E90 centre (46.1162, -23.1463) end of major axis (47.2738, -21.3241) minor radius 1.4234 (44.6084, -24.5806) -> (44.9195, -24.9422) ccw
  ellipse E91 centre (44.5452, -21.3362) end of major axis (43.7632, -17.6184) minor radius 1.1937 (44.9195, -24.9422) -> (45.3157, -25.0563) ccw
  spline S680 degree 3 poles (45.3157, -25.0563) (45.4524, -25.032) (45.5636, -24.9177) (45.6057, -24.7368) knots 2 2 2 2 3 3 3 3
  spline S681 degree 3 poles (45.6057, -24.7368) (45.6492, -24.5578) (45.6174, -24.3207) (45.5033, -24.1057) knots 3 3 3 3 4 4 4 4
  spline S682 degree 3 poles (45.5033, -24.1057) (45.3945, -23.8851) (45.025, -23.4339) (44.6172, -23.1495) knots 4 4 4 4 5 5 5 5
  spline S683 degree 3 poles (44.6172, -23.1495) (44.2137, -22.8552) (43.7989, -22.7046) (43.7164, -22.8172) knots 5 5 5 5 6 6 6 6
  spline S684 degree 3 poles (43.7164, -22.8172) (43.6328, -22.9292) (43.8718, -23.2675) (44.0979, -23.6423) knots 6 6 6 6 7 7 7 7
  spline S685 degree 3 poles (44.0979, -23.6423) (44.3332, -24.0153) (44.531, -24.424) (44.6084, -24.5806) knots 7 7 7 7 8 8 8 8
  spline S686 degree 3 poles (45.1873, -27.8237) (44.9792, -27.5432) (44.7131, -27.2456) (44.433, -26.9966) knots 0 0 0 0 1 1 1 1
  spline S687 degree 3 poles (44.433, -26.9966) (43.8756, -26.4876) (43.2591, -26.2149) (43.1834, -26.3358) knots 1 1 1 1 2 2 2 2
  spline S688 degree 3 poles (43.1834, -26.3358) (43.1084, -26.4502) (43.529, -26.8996) (43.8943, -27.4681) knots 2 2 2 2 3 3 3 3
  spline S689 degree 3 poles (43.8943, -27.4681) (44.2746, -28.0297) (44.5882, -28.6931) (44.7069, -28.9596) knots 3 3 3 3 4 4 4 4
  ellipse E92 centre (45.0762, -28.3101) end of major axis (44.5308, -26.7284) minor radius 0.587 (44.7069, -28.9596) -> (45.1091, -29.6122) ccw
  spline S690 degree 3 poles (45.1091, -29.6122) (45.2474, -29.7727) (45.39, -29.876) (45.529, -29.8541) knots 5 5 5 5 6 6 6 6
  spline S691 degree 3 poles (45.529, -29.8541) (45.6659, -29.8329) (45.7724, -29.6751) (45.8006, -29.4251) knots 6 6 6 6 7 7 7 7
  spline S692 degree 3 poles (45.8006, -29.4251) (45.8299, -29.1775) (45.7735, -28.8464) (45.6223, -28.5264) knots 7 7 7 7 8 8 8 8
  spline S693 degree 3 poles (45.6223, -28.5264) (45.547, -28.3665) (45.3964, -28.1037) (45.1873, -27.8237) knots 8 8 8 8 9 9 9 9
  line L90 (45.2805, -40.2599) -> (45.3069, -40.179)
  ellipse E93 centre (49.2708, -40.8667) end of major axis (46.8455, -46.2471) minor radius 3.9537 (46.8023, -37.3877) -> (45.3069, -40.179) ccw
  spline S694 degree 3 poles (46.8023, -37.3877) (48.4606, -35.3204) (51.1431, -33.7262) (54.3552, -32.8991) knots 2 2 2 2 3 3 3 3
  line L91 (54.3552, -32.8991) -> (54.4298, -32.8784)
  spline S695 degree 3 poles (54.4298, -32.8784) (54.4599, -32.8702) (54.7705, -32.7902) (54.771, -32.7901) knots 4 4 4 4 5 5 5 5
  line L92 (54.771, -32.7901) -> (55.1929, -32.6806)
  spline S696 degree 3 poles (55.1929, -32.6806) (57.6607, -32.0415) (60.4743, -31.9395) (62.5354, -32.4143) knots 6 6 6 6 7 7 7 7
  ellipse E94 centre (62.0381, -37.2482) end of major axis (56.2116, -34.8014) minor radius 4.7702 (65.6245, -33.8433) -> (62.5354, -32.4143) ccw
  spline S697 degree 3 poles (65.6245, -33.8433) (66.4, -34.4244) (67.4977, -35.4767) (67.3904, -35.8897) (67.358, -36.0144) (67.1607, -36.0663) (67.0009, -36.088) knots 8 8 8 8 9 9 9 10 10 10 10
  spline S698 degree 3 poles (67.0009, -36.088) (66.7997, -36.1154) (66.5906, -36.1279) (66.3882, -36.1402) knots 10 10 10 10 11 11 11 11
  spline S699 degree 3 poles (66.3882, -36.1402) (66.1062, -36.157) (65.8146, -36.1746) (65.5259, -36.2318) knots 11 11 11 11 12 12 12 12
  spline S700 degree 3 poles (65.5259, -36.2318) (63.4714, -36.6395) (61.8652, -37.2395) (60.6152, -38.0661) (59.7286, -38.6523) (58.9087, -39.8105) (59.0759, -41.0764) knots 12 12 12 12 13 13 13 14 14 14 14
  spline S701 degree 3 poles (59.0759, -41.0764) (59.2246, -42.2019) (60.2047, -43.3733) (61.3073, -43.7432) knots 14 14 14 14 15 15 15 15
  spline S702 degree 3 poles (61.3073, -43.7432) (61.6562, -43.8601) (62.0222, -43.9118) (62.3972, -43.9118) (64.7833, -43.9118) (67.5231, -41.8158) (68.3995, -41.0898) knots 15 15 15 15 16 16 16 17 17 17 17
  spline S703 degree 3 poles (68.3995, -41.0898) (68.4392, -41.0571) (68.4846, -41.0134) (68.5337, -40.9657) knots 17 17 17 17 18 18 18 18
  spline S704 degree 3 poles (68.5337, -40.9657) (68.6221, -40.8803) (68.804, -40.6989) (68.8846, -40.7107) knots 18 18 18 18 19 19 19 19
  ellipse E95 centre (68.9208, -40.7873) end of major axis (68.9617, -40.8633) minor radius 0.023 (68.9279, -40.7541) -> (68.8846, -40.7107) ccw
  ellipse E96 centre (64.2382, -52.1399) end of major axis (59.5932, -63.5646) minor radius 1.0032 (68.9294, -41.4816) -> (68.9279, -40.7541) ccw
  ellipse E97 centre (57.2225, -34.7374) end of major axis (66.9543, -45.3673) minor radius 9.0943 (68.048, -44.0127) -> (68.9294, -41.4816) ccw
  spline S705 degree 3 poles (68.048, -44.0127) (66.6097, -46.4506) (63.6594, -48.0251) (60.8846, -47.8409) knots 22 22 22 22 23 23 23 23
  spline S706 degree 3 poles (60.8846, -47.8409) (60.4994, -47.8158) (60.1446, -47.7199) (59.7689, -47.6182) knots 23 23 23 23 24 24 24 24
  spline S707 degree 3 poles (59.7689, -47.6182) (59.5086, -47.5478) (59.2394, -47.475) (58.9605, -47.4286) knots 24 24 24 24 25 25 25 25
  spline S708 degree 3 poles (58.9605, -47.4286) (58.4303, -47.3398) (58.1464, -47.6866) (57.8951, -47.9918) (57.804, -48.1025) (57.7098, -48.217) (57.6071, -48.3073) knots 25 25 25 25 26 26 26 27 27 27 27
  ellipse E98 centre (50.9757, -46.2157) end of major axis (43.0915, -46.6179) minor radius 4.2986 (56.2211, -49.2408) -> (57.6071, -48.3073) ccw
  ellipse E99 centre (53.2558, -44.4662) end of major axis (47.0177, -46.046) minor radius 5.5543 (52.8603, -50.0774) -> (56.2211, -49.2408) ccw
  ellipse E100 centre (51.9012, -48.506) end of major axis (48.555, -47.9831) minor radius 1.5001 (51.1383, -49.8856) -> (52.8603, -50.0774) ccw
  spline S709 degree 3 poles (51.1383, -49.8856) (50.2128, -49.673) (49.2434, -49.2709) (48.0874, -48.62) knots 30 30 30 30 31 31 31 31
  spline S710 degree 3 poles (48.0874, -48.62) (47.4398, -48.2556) (46.7317, -47.8036) (46.5283, -47.0473) knots 31 31 31 31 32 32 32 32
  spline S711 degree 3 poles (46.5283, -47.0473) (46.4956, -46.9255) (46.5287, -46.8881) (46.5396, -46.8759) knots 32 32 32 32 33 33 33 33
  ellipse E101 centre (83.8107, -62.5167) end of major axis (46.5161, -46.9118) minor radius 2.1436 (47.4093, -46.8279) -> (46.5396, -46.8759) ccw
  spline S712 degree 3 poles (47.4093, -46.8279) (48.2364, -46.9437) (48.9855, -46.998) (49.7708, -46.9921) knots 34 34 34 34 35 35 35 35
  ellipse E102 centre (48.397, -44.7282) end of major axis (42.6302, -44.1468) minor radius 2.1995 (49.7708, -46.9921) -> (51.1463, -46.9073) ccw
  spline S713 degree 3 poles (51.1463, -46.9073) (52.2824, -46.7672) (53.1141, -46.4319) (53.6891, -45.8822) knots 36 36 36 36 37 37 37 37
  spline S714 degree 3 poles (53.6891, -45.8822) (54.3448, -45.2544) (54.7224, -44.2905) (54.699, -43.3038) knots 37 37 37 37 38 38 38 38
  line L93 (54.699, -43.3038) -> (54.7188, -43.3273)
  spline S715 degree 3 poles (54.7188, -43.3273) (54.6982, -42.4364) (54.3638, -41.6459) (53.7771, -41.1014) knots 39 39 39 39 40 40 40 40
  spline S716 degree 3 poles (53.7771, -41.1014) (52.6778, -40.0819) (50.8734, -40.2607) (49.2685, -40.5081) knots 40 40 40 40 41 41 41 41
  spline S717 degree 3 poles (49.2685, -40.5081) (48.5259, -40.6232) (47.7665, -40.7977) (46.9473, -41.0415) knots 41 41 41 41 42 42 42 42
  spline S718 degree 3 poles (46.9473, -41.0415) (46.6976, -41.1155) (46.4494, -41.2244) (46.2094, -41.3297) knots 42 42 42 42 43 43 43 43
  spline S719 degree 3 poles (46.2094, -41.3297) (45.8954, -41.4676) (45.5706, -41.6102) (45.2565, -41.6652) knots 43 43 43 43 44 44 44 44
  spline S720 degree 3 poles (45.2565, -41.6652) (45.1414, -41.6853) (45.1113, -41.6503) (45.1014, -41.6387) knots 44 44 44 44 45 45 45 45
  spline S721 degree 3 poles (45.1014, -41.6387) (45.0424, -41.5709) (44.9421, -41.3008) (45.2805, -40.2599) knots 45 45 45 45 46 46 46 46
  spline S722 degree 3 poles (45.041, -40.123) (44.8388, -40.7486) (44.6439, -41.5094) (44.9339, -41.8423) knots 0 0 0 0 1 1 1 1
  spline S723 degree 3 poles (44.9339, -41.8423) (45.0121, -41.9322) (45.1588, -42.0296) (45.4165, -41.9843) knots 1 1 1 1 2 2 2 2
  spline S724 degree 3 poles (45.4165, -41.9843) (45.7726, -41.9212) (46.1169, -41.7695) (46.4499, -41.6226) knots 2 2 2 2 3 3 3 3
  spline S725 degree 3 poles (46.4499, -41.6226) (46.6902, -41.5167) (46.9174, -41.4166) (47.1458, -41.3486) knots 3 3 3 3 4 4 4 4
  spline S726 degree 3 poles (47.1458, -41.3486) (47.9495, -41.1081) (48.6935, -40.936) (49.4199, -40.8224) knots 4 4 4 4 5 5 5 5
  spline S727 degree 3 poles (49.4199, -40.8224) (50.9428, -40.5849) (52.6504, -40.408) (53.6356, -41.3187) knots 5 5 5 5 6 6 6 6
  spline S728 degree 3 poles (53.6356, -41.3187) (54.1529, -41.7967) (54.4489, -42.4977) (54.469, -43.2924) knots 6 6 6 6 7 7 7 7
  spline S729 degree 3 poles (54.469, -43.2924) (54.4912, -44.1815) (54.1555, -45.0476) (53.5709, -45.6087) knots 7 7 7 7 8 8 8 8
  spline S730 degree 3 poles (53.5709, -45.6087) (53.0536, -46.1047) (52.2881, -46.4101) (51.2303, -46.5423) (50.781, -46.5984) (50.2998, -46.6282) (49.7999, -46.6308) knots 8 8 8 8 9 9 9 10 10 10 10
  spline S731 degree 3 poles (49.7999, -46.6308) (49.0302, -46.6378) (48.2987, -46.5842) (47.482, -46.4704) knots 10 10 10 10 11 11 11 11
  spline S732 degree 3 poles (47.482, -46.4704) (47.178, -46.4276) (46.5453, -46.3382) (46.2805, -46.637) knots 11 11 11 11 12 12 12 12
  spline S733 degree 3 poles (46.2805, -46.637) (46.2032, -46.7245) (46.1252, -46.8816) (46.1929, -47.1337) knots 12 12 12 12 13 13 13 13
  spline S734 degree 3 poles (46.1929, -47.1337) (46.4206, -47.9799) (47.1575, -48.4934) (47.9199, -48.9223) knots 13 13 13 13 14 14 14 14
  spline S735 degree 3 poles (47.9199, -48.9223) (49.106, -49.59) (50.1055, -50.0037) (51.0647, -50.224) knots 14 14 14 14 15 15 15 15
  ellipse E103 centre (51.8032, -49.1752) end of major axis (48.7665, -48.7006) minor radius 1.1704 (51.0647, -50.224) -> (52.8674, -50.4247) ccw
  spline S736 degree 3 poles (52.8674, -50.4247) (54.087, -50.4157) (55.3036, -50.113) (56.3857, -49.5492) (56.9433, -49.2587) (57.4325, -48.9292) (57.8399, -48.5702) knots 16 16 16 16 17 17 17 18 18 18 18
  spline S737 degree 3 poles (57.8399, -48.5702) (57.9637, -48.4612) (58.0672, -48.3356) (58.1672, -48.2141) knots 18 18 18 18 19 19 19 19
  spline S738 degree 3 poles (58.1672, -48.2141) (58.4193, -47.9077) (58.5914, -47.7223) (58.9025, -47.7746) knots 19 19 19 19 20 20 20 20
  spline S739 degree 3 poles (58.9025, -47.7746) (59.1638, -47.8182) (59.4244, -47.8886) (59.6765, -47.9568) knots 20 20 20 20 21 21 21 21
  spline S740 degree 3 poles (59.6765, -47.9568) (60.0523, -48.0585) (60.4411, -48.1636) (60.861, -48.191) knots 21 21 21 21 22 22 22 22
  spline S741 degree 3 poles (60.861, -48.191) (63.8145, -48.3857) (66.8245, -46.7786) (68.3515, -44.1901) (68.809, -43.4146) (69.1203, -42.5221) (69.2767, -41.5376) knots 22 22 22 22 23 23 23 24 24 24 24
  spline S742 degree 3 poles (69.2767, -41.5376) (69.3334, -41.1822) (69.3711, -40.7883) (69.2216, -40.561) knots 24 24 24 24 25 25 25 25
  spline S743 degree 3 poles (69.2216, -40.561) (69.1241, -40.4132) (69.0047, -40.3714) (68.9219, -40.3623) knots 25 25 25 25 26 26 26 26
  spline S744 degree 3 poles (68.9219, -40.3623) (68.6814, -40.3348) (68.4616, -40.5458) (68.2871, -40.7147) knots 26 26 26 26 27 27 27 27
  spline S745 degree 3 poles (68.2871, -40.7147) (68.2453, -40.7552) (68.207, -40.7927) (68.1734, -40.8205) (67.1945, -41.6312) (63.8147, -44.214) (61.4183, -43.4109) knots 27 27 27 27 28 28 28 29 29 29 29
  spline S746 degree 3 poles (61.4183, -43.4109) (60.4492, -43.0857) (59.5548, -42.0188) (59.4244, -41.0324) knots 29 29 29 29 30 30 30 30
  spline S747 degree 3 poles (59.4244, -41.0324) (59.2773, -39.9176) (60.0137, -38.8882) (60.8089, -38.3625) (62.02, -37.5618) (63.5851, -36.9789) (65.5936, -36.5804) knots 30 30 30 30 31 31 31 32 32 32 32
  spline S748 degree 3 poles (65.5936, -36.5804) (65.8588, -36.5278) (66.1258, -36.5117) (66.4085, -36.4948) knots 32 32 32 32 33 33 33 33
  spline S749 degree 3 poles (66.4085, -36.4948) (66.6173, -36.4823) (66.8333, -36.4693) (67.0476, -36.4401) knots 33 33 33 33 34 34 34 34
  ellipse E104 centre (54.5644, -28.2771) end of major axis (41.4536, -20.4391) minor radius 2.7399 (67.0476, -36.4401) -> (67.7309, -35.981) ccw
  spline S750 degree 3 poles (67.7309, -35.981) (67.9418, -35.1698) (66.0514, -33.7255) (65.8351, -33.5634) knots 35 35 35 35 36 36 36 36
  ellipse E105 centre (62.1029, -37.1208) end of major axis (56.0301, -34.5597) minor radius 4.9766 (65.8351, -33.5634) -> (62.621, -32.0767) ccw
  spline S751 degree 3 poles (62.621, -32.0767) (61.7364, -31.873) (60.7182, -31.7727) (59.6482, -31.7727) (58.1618, -31.7727) (56.5757, -31.9664) (55.1108, -32.3457) knots 37 37 37 37 38 38 38 39 39 39 39
  line L94 (55.1108, -32.3457) -> (54.6835, -32.4565)
  spline S752 degree 3 poles (54.6835, -32.4565) (54.5073, -32.5019) (54.403, -32.5288) (54.339, -32.5505) knots 40 40 40 40 41 41 41 41
  line L95 (54.339, -32.5505) -> (54.3378, -32.546)
  spline S753 degree 3 poles (54.3378, -32.546) (51.0535, -33.3965) (48.3069, -35.0373) (46.604, -37.1659) knots 42 42 42 42 43 43 43 43
  ellipse E106 centre (49.148, -40.7618) end of major axis (51.6727, -35.1479) minor radius 4.0732 (46.604, -37.1659) -> (45.0558, -40.0766) ccw
  line L96 (45.0558, -40.0766) -> (45.041, -40.123)
  spline S754 degree 3 poles (50.5737, -43.0887) (50.887, -43.0079) (51.2072, -43.1962) (51.2883, -43.5098) knots 0 0 0 0 1 1 1 1
  spline S755 degree 3 poles (51.2883, -43.5098) (51.3696, -43.8231) (51.1813, -44.1429) (50.8677, -44.2245) knots 1 1 1 1 2 2 2 2
  spline S756 degree 3 poles (50.8677, -44.2245) (50.5541, -44.3054) (50.2342, -44.117) (50.1529, -43.8034) knots 2 2 2 2 3 3 3 3
  spline S757 degree 3 poles (50.1529, -43.8034) (50.0718, -43.4898) (50.2599, -43.17) (50.5737, -43.0887) knots 3 3 3 3 4 4 4 4
  spline S758 degree 3 poles (50.8034, -45.1363) (51.6163, -44.9255) (52.1048, -44.0958) (51.8945, -43.2824) knots 0 0 0 0 1 1 1 1
  spline S759 degree 3 poles (51.8945, -43.2824) (51.6838, -42.469) (50.8536, -41.9808) (50.0407, -42.1912) knots 1 1 1 1 2 2 2 2
  spline S760 degree 3 poles (50.0407, -42.1912) (49.2274, -42.4019) (48.739, -43.2316) (48.9495, -44.0455) knots 2 2 2 2 3 3 3 3
  spline S761 degree 3 poles (48.9495, -44.0455) (49.1602, -44.8584) (49.9903, -45.3466) (50.8034, -45.1363) knots 3 3 3 3 4 4 4 4
  spline S762 degree 3 poles (63.2811, -41.0092) (62.9675, -41.0908) (62.6476, -40.9022) (62.5663, -40.5886) knots 0 0 0 0 1 1 1 1
  spline S763 degree 3 poles (62.5663, -40.5886) (62.4852, -40.2753) (62.6735, -39.9551) (62.9871, -39.8742) knots 1 1 1 1 2 2 2 2
  spline S764 degree 3 poles (62.9871, -39.8742) (63.3002, -39.7926) (63.6206, -39.9813) (63.7015, -40.2949) knots 2 2 2 2 3 3 3 3
  spline S765 degree 3 poles (63.7015, -40.2949) (63.783, -40.6081) (63.5945, -40.9284) (63.2811, -41.0092) knots 3 3 3 3 4 4 4 4
  spline S766 degree 3 poles (63.0976, -38.8101) (62.2846, -39.0204) (61.7959, -39.8501) (62.0066, -40.6635) knots 0 0 0 0 1 1 1 1
  spline S767 degree 3 poles (62.0066, -40.6635) (62.2171, -41.4769) (63.0471, -41.9651) (63.8603, -41.7547) knots 1 1 1 1 2 2 2 2
  spline S768 degree 3 poles (63.8603, -41.7547) (64.6736, -41.544) (65.1621, -40.7143) (64.9514, -39.9009) knots 2 2 2 2 3 3 3 3
  spline S769 degree 3 poles (64.9514, -39.9009) (64.7407, -39.0875) (63.9109, -38.5993) (63.0976, -38.8101) knots 3 3 3 3 4 4 4 4
  spline S770 degree 3 poles (57.5408, -39.5984) (57.592, -39.559) (57.7479, -39.4389) (57.7889, -39.4346) knots 0 0 0 0 1 1 1 1
  spline S771 degree 3 poles (57.7889, -39.4346) (57.8158, -39.4876) (57.7493, -39.7004) (57.6704, -39.8141) knots 1 1 1 1 2 2 2 2
  spline S772 degree 3 poles (57.6704, -39.8141) (57.3772, -40.2364) (56.738, -40.5387) (56.189, -40.5387) (56.1161, -40.5387) (56.045, -40.5334) (55.9764, -40.5223) knots 2 2 2 2 3 3 3 4 4 4 4
  line L97 (55.9764, -40.5223) -> (55.9383, -40.5163)
  spline S773 degree 3 poles (55.9383, -40.5163) (55.7323, -40.4835) (55.4209, -40.4339) (55.3653, -40.2664) knots 5 5 5 5 6 6 6 6
  spline S774 degree 3 poles (55.3653, -40.2664) (55.3846, -40.2448) (55.4686, -40.1832) (55.8143, -40.1405) knots 6 6 6 6 7 7 7 7
  line L98 (55.8143, -40.1405) -> (55.9881, -40.1183)
  spline S775 degree 3 poles (55.9881, -40.1183) (56.5058, -40.0526) (56.9946, -39.9906) (57.4738, -39.649) knots 8 8 8 8 9 9 9 9
  spline S776 degree 3 poles (57.4738, -39.649) (57.4933, -39.6351) (57.5159, -39.6177) (57.5408, -39.5984) knots 9 9 9 9 10 10 10 10
  spline S777 degree 3 poles (56.0145, -37.6481) (54.9218, -37.9313) (54.3102, -39.2191) (54.5176, -40.0196) knots 0 0 0 0 1 1 1 1
  spline S778 degree 3 poles (54.5176, -40.0196) (54.7249, -40.8205) (55.7788, -41.24) (56.8712, -40.9571) knots 1 1 1 1 2 2 2 2